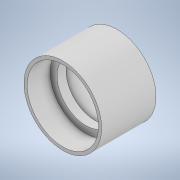
# Autodesk Inventor part: Roller
Saved by Autodesk Inventor 2021 (Build 250183000, 183)
## iProperties
Created: 2021-02-26
Part Number: Roller
Material: Generic
Document SubType Name: Modeling
Designer: Viktor
Density: 1 g/cm^3
Appearance: Default
Author: Viktor
## iProperties of the stored document _3DPrint.ipt
Created: 2021-02-26
Part Number: _3DPrint
Material: Generic
Document SubType Name: Modeling
Designer: Viktor
Density: 1 g/cm^3
Appearance: Default
Author: Viktor
Autodesk Inventor part; units mm, degrees
ref_plane "YZ Plane" through (0, 0, 0) normal (1, 0, 0) x (0, 1, 0)
ref_plane "XZ Plane" through (0, 0, 0) normal (0, 1, 0) x (-1, 0, 0)
sketch "Sketch1" plane through (0, 0, 0) normal (0, 0, 1) x (1, 0, 0)
  circle A0 centre (0, 0) radius 12.15
  dimension "d0" = 24.3
  constraints: 1 centre point, 1 coincident
  measures "d0" diameter of A0
extrude "Extrusion1" add sketch "Sketch1" along normal blind 17
sketch "Sketch2" plane through (0, 0, 17) normal (0, 0, 1) x (1, 0, 0)
  circle A0 centre (0, 0) radius 11.15
  dimension "d3" = 22.3
  constraints: 1 centre point, 1 coincident
  measures "d3" diameter of A0
extrude "Extrusion2" cut sketch "Sketch2" against normal blind 20
ref_plane "Work Plane1" through (0, 0, 7) normal (0, 0, -1) x (-1, 0, 0)
sketch "Sketch3" plane through (0, 0, 7) normal (0, 0, -1) x (-1, 0, 0)
  circle A0 centre (0, 0) radius 11.15 projected
  circle A1 centre (0, 0) radius 9
  dimension "d7" = 18
  constraints: 1 centre point, 1 coincident
  measures "d7" diameter of A1
extrude "Extrusion3" add sketch "Sketch3" against normal blind 2.8
body "Solid1"
